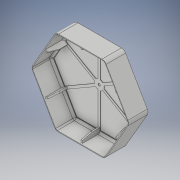
# Autodesk Inventor part: Base v3
Saved by Autodesk Inventor 2019 (Build 230136000, 136)
## iProperties
Created: 2021-07-14
Part Number: Base v3
Material: Generic
Document SubType Name: Modeling
Designer: Lix
Density: 1 g/cm^3
Appearance: Default
Author: Lix
Autodesk Inventor part; units mm, degrees
ref_plane "YZ Plane" through (0, 0, 0) normal (1, 0, 0) x (0, 1, 0)
ref_plane "XZ Plane" through (0, 0, 0) normal (0, 1, 0) x (-1, 0, 0)
ref_plane "XY Plane" through (0, 0, 0) normal (0, 0, 1) x (1, 0, 0)
sketch "Sketch1" plane through (0, 0, 0) normal (0, 0, 1) x (1, 0, 0)
  line L0 (50.5181, -87.5) -> (-50.5181, -87.5)
  line L1 (-50.5181, -87.5) -> (-101.0363, 0)
  line L2 (-101.0363, 0) -> (-50.5181, 87.5)
  line L3 (-50.5181, 87.5) -> (50.5181, 87.5)
  line L4 (50.5181, 87.5) -> (101.0363, 0)
  line L5 (101.0363, 0) -> (50.5181, -87.5)
  point P0 (0, 0)
  point P1 (0, 0)
  point P2 (0, 0)
  dimension "d0" = 175
  constraints: 12 end point, 2 coincident, 1 horizontal, 13 other
  measures "d0" distance between parallel lines of L5 L2
extrude "Extrusion1" add sketch "Sketch1" along normal blind 40
shell "Shell1" thickness 1.5 removed faces 1 at (16.8394, -29.1667, 40) ; own thickness 1 on faces at (16.8394, -29.1667, 0)
ref_plane "Work Plane1" through (-25.2591, 43.75, 40) normal (0.8660254, 0.5, 0) x (0, 0, -1)
ref_plane "Work Plane2" through (-50.5181, 0, 0) normal (0, 1, 0) x (1, 0, 0)
ref_plane "Work Plane3" through (-25.2591, -43.75, 0) normal (-0.8660254, 0.5, 0) x (0, 0, 1)
sketch "Sketch4" plane through (-49.6521, -86, 1) normal (0, 0, 1) x (1, 0, 0)
  line L0 (99.3042, 0) -> (0, 0) projected
  line L1 (148.9564, 86) -> (99.3042, 0) projected
  line L2 (99.3042, 172) -> (148.9564, 86) projected
  line L3 (0, 172) -> (99.3042, 172) projected
  line L4 (-49.6521, 86) -> (0, 172) projected
  line L5 (0, 0) -> (-49.6521, 86) projected
  line L6 (-19.2831, 128.6007) -> (2.8868, 167)
  line L7 (2.8868, 167) -> (47.2265, 167)
  line L8 (99.3042, 172) -> (0, 0) construction
  arc A0 (47.2265, 95.7014) -> (42.4633, 92.9514) centre (49.6521, 86) ccw
  line L9 (-19.2831, 128.6007) -> (42.4633, 92.9514)
  line L10 (47.2265, 167) -> (47.2265, 95.7014)
  circle A1 centre (49.6521, 86) radius 2.5
  arc A2 (40.0377, 88.75) -> (40.0377, 83.25) centre (49.6521, 86) ccw
  line L11 (-21.7088, 124.3993) -> (40.0377, 88.75)
  line L12 (-21.7088, 47.6007) -> (40.0377, 83.25)
  line L13 (-21.7088, 47.6007) -> (-43.8786, 86)
  line L14 (-43.8786, 86) -> (-21.7088, 124.3993)
  arc A3 (42.4633, 79.0486) -> (47.2265, 76.2986) centre (49.6521, 86) ccw
  line L15 (-19.2831, 43.3993) -> (42.4633, 79.0486)
  line L16 (47.2265, 5) -> (47.2265, 76.2986)
  line L17 (47.2265, 5) -> (2.8868, 5)
  line L18 (2.8868, 5) -> (-19.2831, 43.3993)
  arc A4 (52.0778, 76.2986) -> (56.8409, 79.0486) centre (49.6521, 86) ccw
  line L19 (52.0778, 5) -> (52.0778, 76.2986)
  line L20 (118.5874, 43.3993) -> (56.8409, 79.0486)
  line L21 (118.5874, 43.3993) -> (96.4175, 5)
  line L22 (96.4175, 5) -> (52.0778, 5)
  arc A5 (59.2666, 83.25) -> (59.2666, 88.75) centre (49.6521, 86) ccw
  line L23 (121.013, 47.6007) -> (59.2666, 83.25)
  line L24 (121.013, 124.3993) -> (59.2666, 88.75)
  line L25 (121.013, 124.3993) -> (143.1829, 86)
  line L26 (143.1829, 86) -> (121.013, 47.6007)
  arc A6 (56.8409, 92.9514) -> (52.0778, 95.7014) centre (49.6521, 86) ccw
  line L27 (118.5874, 128.6007) -> (56.8409, 92.9514)
  line L28 (52.0778, 167) -> (52.0778, 95.7014)
  line L29 (52.0778, 167) -> (96.4175, 167)
  line L30 (96.4175, 167) -> (118.5874, 128.6007)
  point P0 (-49.6521, 86)
  point P1 (0, 0)
  point P2 (99.3042, 0)
  point P3 (148.9564, 86)
  point P4 (99.3042, 172)
  dimension "d37" = 5
  dimension "d44" = 10
  dimension "d45" = 60
  dimension "d46" = 90
  dimension "d47" = 90
  dimension "d52" = 5.5
  dimension "d55" = 5
  dimension "d72" = 360
  constraints: 50 end point, 12 point on circle, 7 centre point, 2 equal length, 1 coincident, 1 midpoint, 73 other
  measures "d37" distance between parallel lines of L3 L7
  measures "d44" radius of A0
  measures "d45" angle of L10 L9
  measures "d46" angle of L9 L6
  measures "d47" angle of L10 L7
  measures "d52" distance of L10.end L9.end
  measures "d55" diameter of A1
extrude "Extrusion5" cut sketch "Sketch4" against normal blind 0.75 contours L6 L7 L10 A0 L9 | A1 | A2 L12 L13 L14 L11 | A3 L16 L17 L18 L15 | A4 L20 L21 L22 L19 | A5 L24 L25 L26 L23 | A6 L28 L29 L30 L27
sketch "Sketch8" plane through (-49.6521, -86, 1) normal (0, 0, 1) x (1, 0, 0)
  line L0 (99.3042, 0) -> (0, 0) projected
  line L1 (148.9564, 86) -> (99.3042, 0) projected
  line L2 (99.3042, 172) -> (148.9564, 86) projected
  line L3 (0, 172) -> (99.3042, 172) projected
  line L4 (-49.6521, 86) -> (0, 172) projected
  line L5 (0, 0) -> (-49.6521, 86) projected
  line L6 (48.1521, 162) -> (51.1521, 162)
  line L7 (51.1521, 162) -> (51.1521, 172)
  line L8 (51.1521, 172) -> (48.1521, 172)
  line L9 (48.1521, 172) -> (48.1521, 162)
  line L10 (0, 172) -> (99.3042, 172) projected
  line L11 (49.6521, 86) -> (49.6521, 172)
  point P0 (49.6521, 86)
  point P1 (49.6521, 172)
  dimension "d57" = 3
  dimension "d58" = 10
  constraints: 10 end point, 2 midpoint, 2 parallel, 1 coincident, 1 collinear, 1 horizontal, 1 perpendicular, 1 vertical
  measures "d57" distance of L6.start L6.end
  measures "d58" distance of L6.end L7.end
extrude "Extrusion6" add sketch "Sketch8" along normal blind 36 contours L7 L6 L11 L3 | L3 L11 L6 L9
sketch "Sketch9" plane through (1.5, 76, 1) normal (1, 0, 0) x (0, 0, -1)
  line L0 (0, 0) -> (0, 10) projected
  line L1 (0, 0) -> (-36, 0) projected
  line L2 (-36, 10) -> (-36, 0) projected
  line L3 (0, 10) -> (-36, 10) projected
  line L4 (-36, 10) -> (-36, 0) projected
  line L5 (-36, 0) -> (-16, 0)
  line L6 (0, 0) -> (-36, 0) projected
  line L7 (-16, 0) -> (-36, 5)
  line L8 (-36, 5) -> (-36, 0)
  point P0 (1, -76)
  point P1 (-36, 8)
  dimension "d77" = 5
  dimension "d78" = 20
  constraints: 6 end point, 3 point on line, 1 collinear, 1 perpendicular
  measures "d77" distance of L7.end L5.start
  measures "d78" distance of L5.start L5.end
extrude "Extrusion8" cut sketch "Sketch9" against normal blind 20 contours L1 L2 L7
pattern_circular "Circular Pattern1" count 6 over 360 about axis through (0, 0, 1) along (0, 0, -1) of "Extrusion6", "Extrusion8"
fillet "Fillet1" radius 4 18 edges at (-25.5761, -86, 1) (25.5761, -86, 1) (-87.2662, -20.8505, 1) (-61.6902, -65.1495, 1) (61.6902, -65.1495, 1) (87.2662, -20.8505, 1) (87.2662, 20.8505, 1) (61.6902, 65.1495, 1) (25.5761, 86, 1) (-25.5761, 86, 1) (-61.6902, 65.1495, 1) (-87.2662, 20.8505, 1) (-99.3042, 0, 20.5) (-49.6521, 86, 20.5) (49.6521, 86, 20.5) (99.3042, 0, 20.5) (49.6521, -86, 20.5) (-49.6521, -86, 20.5)
fillet "Fillet2" radius 10 6 edges at (101.0363, 0, 20) (50.5181, 87.5, 20) (-50.5181, 87.5, 20) (50.5181, -87.5, 20) (-101.0363, 0, 20) (-50.5181, -87.5, 20)
fillet "Fillet4" radius 2 5 edges at (-7.1888, 6.9514, 0.625) (-2.4257, 9.7014, 0.625) (-2.4257, 81, 0.625) (-46.7654, 81, 0.625) (-68.9352, 42.6007, 0.625)
sketch "Sketch5" plane through (-44.7446, 87.5, 0) normal (0, 1, 0) x (1, 0, 0)
  line L0 (0, 0) -> (89.4893, 0) projected
  line L1 (0, -40) -> (0, 0) projected
  point P0 (44.7446, 0)
  point P1 (44.7446, -20)
  point P2 (44.7446, 0)
  point P3 (0, -20)
  constraints: 2 midpoint, 1 horizontal alignment, 1 vertical alignment
sketch "Sketch6" plane through (53.4049, 82.5, 40) normal (0.8660254, 0.5, 0) x (0, 0, -1)
  line L0 (40, 8.6603) -> (0, 8.6603) projected
  point P0 (40, -44.7446)
  point P1 (20, -44.7446)
  point P2 (20, 8.6603)
  constraints: 1 horizontal alignment, 1 midpoint, 1 vertical alignment
sketch "Sketch7" plane through (53.4049, -82.5, 40) normal (0.8660254, -0.5, 0) x (0, 0, -1)
  line L0 (0, -8.6603) -> (40, -8.6603) projected
  point P0 (40, 44.7446)
  point P1 (20, 44.7446)
  point P2 (20, -8.6603)
  constraints: 1 horizontal alignment, 1 midpoint, 1 vertical alignment
body "Solid1"
